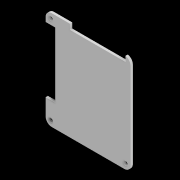
# Autodesk Inventor part: ArducamHat
Saved by Autodesk Inventor 2020 (Build 240168000, 168)
## iProperties
Created: 2020-11-17
Part Number: ArducamHat
Material: Generic
Document SubType Name: Modeling
Designer: valer
Density: 1 g/cm^3
Appearance: Default
Author: valer
Autodesk Inventor part; units mm, degrees
ref_plane "YZ Plane" through (0, 0, 0) normal (1, 0, 0) x (0, 1, 0)
ref_plane "XZ Plane" through (0, 0, 0) normal (0, 1, 0) x (-1, 0, 0)
ref_plane "XY Plane" through (0, 0, 0) normal (0, 0, 1) x (1, 0, 0)
sketch "Base" plane through (0, 0, 0) normal (0, 0, 1) x (1, 0, 0)
  line L0 (-24, 32.5) -> (24, 32.5)
  line L1 (28, 28.5) -> (28, -28.5)
  line L2 (24, -32.5) -> (-24, -32.5)
  line L3 (-28, -28.5) -> (-28, 28.5)
  line L4 (-24.6441, 29) -> (24.6441, 29)
  line L5 (24.6441, 29) -> (24.6441, -29)
  line L6 (24.6441, -29) -> (-24.6441, -29)
  line L7 (-24.6441, -29) -> (-24.6441, 29)
  line L8 (-24.6441, 29) -> (24.6441, -29)
  line L9 (24.6441, 29) -> (-24.6441, -29)
  line L10 (-12, 29) -> (-12, 32.5)
  line L11 (24.6441, 29) -> (24.6441, 32.5)
  circle A0 centre (24.6441, -29) radius 1.38
  circle A1 centre (-24.6441, 29) radius 1.38
  circle A2 centre (-24.6441, -29) radius 1.38
  line L12 (-28, 25.5) -> (-21.65, 25.5)
  line L13 (-21.65, 25.5) -> (-21.65, -17.5)
  line L14 (-21.65, -17.5) -> (-28, -17.5)
  line L15 (-28, -17.5) -> (-28, 25.5)
  line L16 (-9.2839, 21.1377) -> (1.8117, 21.1377)
  line L17 (1.8117, 21.1377) -> (1.8117, 18.6377)
  line L18 (1.8117, 18.6377) -> (-9.2839, 18.6377)
  line L19 (-9.2839, 18.6377) -> (-9.2839, 21.1377)
  line L20 (9.5485, 21.1377) -> (20.6441, 21.1377)
  line L21 (20.6441, 21.1377) -> (20.6441, 18.6377)
  line L22 (20.6441, 18.6377) -> (9.5485, 18.6377)
  line L23 (9.5485, 18.6377) -> (9.5485, 21.1377)
  line L24 (21.5345, 10.4789) -> (24.0345, 10.4789)
  line L25 (24.0345, 10.4789) -> (24.0345, -0.6167)
  line L26 (24.0345, -0.6167) -> (21.5345, -0.6167)
  line L27 (21.5345, -0.6167) -> (21.5345, 10.4789)
  line L28 (21.5345, -8.4887) -> (24.0345, -8.4887)
  line L29 (24.0345, -8.4887) -> (24.0345, -19.5843)
  line L30 (24.0345, -19.5843) -> (21.5345, -19.5843)
  line L31 (21.5345, -19.5843) -> (21.5345, -8.4887)
  line L32 (-14.8613, -28.3904) -> (-3.7657, -28.3904)
  line L33 (-3.7657, -28.3904) -> (-3.7657, -25.8904)
  line L34 (-3.7657, -25.8904) -> (-14.8613, -25.8904)
  line L35 (-14.8613, -25.8904) -> (-14.8613, -28.3904)
  line L36 (4.2175, -25.8904) -> (15.3131, -25.8904)
  line L37 (15.3131, -25.8904) -> (15.3131, -28.3904)
  line L38 (15.3131, -28.3904) -> (4.2175, -28.3904)
  line L39 (4.2175, -28.3904) -> (4.2175, -25.8904)
  arc A3 (-24, 32.5) -> (-28, 28.5) centre (-24, 28.5) ccw
  arc A4 (28, 28.5) -> (24, 32.5) centre (24, 28.5) ccw
  arc A5 (24, -32.5) -> (28, -28.5) centre (24, -28.5) ccw
  arc A6 (-28, -28.5) -> (-24, -32.5) centre (-24, -28.5) ccw
  point P0 (0, 0)
  point P1 (-28, 32.5)
  point P2 (28, 32.5)
  point P3 (-28, -32.5)
  point P4 (0, 0)
  point P5 (-21.65, 25.4766)
  point P6 (24.6441, 32.4478)
  point P7 (-21.6699, 25.5)
  dimension "d0" = 56
  dimension "d1" = 65
  dimension "d2" = 58
  dimension "d3" = 3.3559
  dimension "d4" = 3.3559
  dimension "d5" = 3.5
  dimension "d6" = 3.5
  dimension "d7" = 16
  dimension "d8" = 2.76
  dimension "d9" = 6.35
  dimension "d10" = 3.5
  dimension "d11" = 43
  dimension "d12" = 2.5
  dimension "d13" = 4
  dimension "d14" = 0.6096
  dimension "d15" = 0.6096
  dimension "d16" = 4
  dimension "d17" = 49.2883
  dimension "d18" = 18.7161
  dimension "d19" = 7.7369
  dimension "d20" = 7.9832
  dimension "d21" = 7.872
  dimension "d22" = 12.9157
  dimension "d23" = 13.1387
  dimension "d24" = 7.8623
  constraints: 80 end point, 18 parallel, 11 perpendicular, 11 point on line, 10 equal length, 9 horizontal, 8 point on circle, 8 tangent, 7 centre point, 5 equal radius, 4 coincident, 2 collinear, 1 midpoint
  measures "d0" distance of point (-28, 32.5) point (28, 32.5)
  measures "d1" distance of point (-28, -32.5) point (-28, 32.5)
  measures "d2" distance of L6.end L4.start
  measures "d3" distance between parallel lines of L3 L7
  measures "d4" distance between parallel lines of L1 L5
  measures "d5" distance between parallel lines of L0 L4
  measures "d6" distance between parallel lines of L2 L6
  measures "d7" distance between parallel lines of L3 L10
  measures "d8" diameter of A0
  measures "d9" distance between parallel lines of L15 L13
  measures "d10" distance between parallel lines of L12 L4
  measures "d11" distance between parallel lines of L14 L12
  measures "d12" distance of L18.end L16.start
  measures "d13" distance between parallel lines of L5 L21
  measures "d14" distance between parallel lines of L5 L25
  measures "d15" distance between parallel lines of L6 L38
  measures "d16" radius of A3
  measures "d17" distance between parallel lines of L7 L5
  measures "d18" distance between parallel lines of L15 L19
  measures "d19" distance between parallel lines of L23 L17
  measures "d20" distance between parallel lines of L39 L33
  measures "d21" distance between parallel lines of L26 L28
  measures "d22" distance between parallel lines of L2 L30
  measures "d23" distance between parallel lines of L3 L35
  measures "d24" distance between parallel lines of L4 L16
extrude "BaseFeature" add sketch "Base" along normal blind 1.5 contours L0 L10 L4 A1 L7 L12 L3 A3 | L4 L9 L20 L23 L22 L8 L13 L12 A1 | A4 L1 A5 L2 A6 L3 L14 L7 A2 L6 A0 L5 L11 | L5 A0 L8 L9 L22 L21 L20 | L7 A1 L8 L12 | L20 L21 L22 L9 | L9 L22 L23 L20 | L14 L13 L8 L9 A2 L7 | L12 L13 L8 | A0 L6 A2 L9 L8 | L16 L17 L18 L19 | L24 L25 L26 L27 | L28 L29 L30 L31 | L35 L34 L33 L32 | L36 L37 L38 L39
extrude "ConnectorsFeature" add sketch "Base" against normal blind 1 contours L20 L21 L22 L9 | L9 L22 L23 L20 | L16 L17 L18 L19 | L24 L25 L26 L27 | L28 L29 L30 L31 | L35 L34 L33 L32 | L36 L37 L38 L39
equation "\"d4\" = d3"
equation "\"d6\" = d5"
equation "\"d10\" = d5"
body "Solid1"
